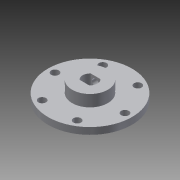
# Autodesk Inventor part: Snow Blower Hub
Saved by Autodesk Inventor 2013 (Build 170138000, 138)
## iProperties
Created: 2013-01-18
Part Number: Snow Blower Hub
Material: Aluminum 6061
Document SubType Name: Modeling
Designer: actoennies
Density: 2.71 g/cm^3
Mass: 37.4819 g
Surface Area: 71.0733 cm^2
Volume: 13.831 cm^3
Author: actoennies
Autodesk Inventor part; units mm, degrees
ref_plane "YZ Plane" through (0, 0, 0) normal (1, 0, 0) x (0, 1, 0)
ref_plane "XZ Plane" through (0, 0, 0) normal (0, 1, 0) x (-1, 0, 0)
ref_plane "XY Plane" through (0, 0, 0) normal (0, 0, 1) x (1, 0, 0)
sketch "Sketch1" plane through (0, 0, 0) normal (0, 1, 0) x (-1, 0, 0)
  circle A0 centre (0, 0) radius 28.575
  circle A1 centre (0, 0) radius 23.8125 construction
  circle A2 centre (23.8125, 0) radius 2.5908
  circle A3 centre (0, 0) radius 28.575
  circle A4 centre (11.9063, 20.6222) radius 2.5908
  circle A5 centre (0, 0) radius 28.575
  circle A6 centre (-11.9062, 20.6222) radius 2.5908
  circle A7 centre (0, 0) radius 28.575
  circle A8 centre (-23.8125, 0) radius 2.5908
  circle A9 centre (0, 0) radius 28.575
  circle A10 centre (-11.9063, -20.6222) radius 2.5908
  circle A11 centre (0, 0) radius 28.575
  circle A12 centre (11.9062, -20.6222) radius 2.5908
  line L0 (-3.3001, 3.7528) -> (3.3001, 3.7528)
  line L1 (-3.3001, -3.7528) -> (3.3001, -3.7528)
  arc A13 (-3.3001, 3.7528) -> (-3.3001, -3.7528) centre (0, 0) ccw
  arc A14 (3.3001, -3.7528) -> (3.3001, 3.7528) centre (0, 0) ccw
  dimension "d1" = 47.625
  dimension "d0" = 57.15
  dimension "d2" = 5.1816
  dimension "d5" = 360
  dimension "d8" = 7.5057
  dimension "d9" = 3.7529
  constraints: 14 centre point, 5 coincident, 4 end point, 4 point on circle, 1 horizontal, 1 horizontal alignment, 1 parallel, 25 other
  measures "d0" diameter of A0
  measures "d2" diameter of A2
  measures "d8" distance between parallel lines of L0 L1
  measures "d9" distance from line of L0 point (0, 0)
extrude "Extrusion1" add sketch "Sketch1" along normal blind 4.572
sketch "Sketch2" plane through (0, 4.572, 0) normal (0, 1, 0) x (1, 0, 0)
  arc A0 (-3.3001, 3.7528) -> (-3.3001, -3.7528) centre (0, 0) ccw projected
  line L0 (-3.3001, 3.7528) -> (3.3001, 3.7528) projected
  arc A1 (3.3001, -3.7528) -> (3.3001, 3.7528) centre (0, 0) ccw projected
  line L1 (3.3001, -3.7528) -> (-3.3001, -3.7528) projected
  circle A2 centre (0, 0) radius 28.575 projected
  circle A3 centre (0, 0) radius 12.1666
  dimension "d12" = 24.3332
  constraints: 1 centre point, 1 coincident
  measures "d12" diameter of A3
extrude "Extrusion2" add sketch "Sketch2" along normal blind 7.874 contours A3
sketch "Sketch3" plane through (-3.3001, 0, -3.7528) normal (0, 0, 1) x (1, 0, 0)
  line L0 (6.6002, 0) -> (6.6002, 12.446) projected
  line L1 (0, 12.446) -> (6.6002, 12.446) projected
  circle A0 centre (3.3001, 8.636) radius 2.413
  point P0 (3.3001, 0)
  dimension "d16" = 4.826
  dimension "d17" = 3.81
  dimension "d18" = 3.3001
  constraints: 1 centre point
  measures "d16" diameter of A0
  measures "d17" distance from line of L1 A0.centre
  measures "d18" distance from line of L0 A0.centre
extrude "Extrusion3" cut sketch "Sketch3" against normal blind 7.874
equation "\"d9\" = 0.5 * d8"
body "Solid1"
